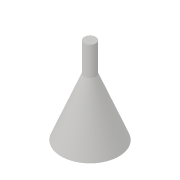
# Autodesk Inventor part: control stick
Saved by Autodesk Inventor 2018 (Build 220112000, 112)
## iProperties
Created: 2019-02-02
Part Number: control stick
Material: Generic
Document SubType Name: Modeling
Designer: ball
Density: 1 g/cm^3
Appearance: Default
Author: ball
Autodesk Inventor part; units mm, degrees
ref_plane "YZ Plane" through (0, 0, 0) normal (1, 0, 0) x (0, 1, 0)
ref_plane "XZ Plane" through (0, 0, 0) normal (0, 1, 0) x (-1, 0, 0)
ref_plane "XY Plane" through (0, 0, 0) normal (0, 0, 1) x (1, 0, 0)
sketch "Sketch1" plane through (0, 0, 0) normal (0, 0, 1) x (1, 0, 0)
  line L0 (0, 0) -> (12.7, 0)
  line L1 (0, 0) -> (0, 25.4)
  line L2 (0, 25.4) -> (2.54, 25.4)
  line L3 (2.54, 25.4) -> (12.7, 0)
  line L4 (0, 25.4) -> (2.54, 25.4)
  line L5 (2.54, 25.4) -> (2.54, 38.1)
  line L6 (2.54, 38.1) -> (0, 38.1)
  line L7 (0, 38.1) -> (0, 25.4)
  dimension "d0" = 12.7
  dimension "d1" = 25.4
  dimension "d2" = 2.54
  dimension "d3" = 12.7
  constraints: 16 end point, 3 horizontal, 2 parallel, 1 perpendicular, 1 vertical
  measures "d0" distance of L0.start L0.end
  measures "d1" distance of L0.start L1.end
  measures "d2" distance of L1.end L2.end
  measures "d3" distance of L5.end L4.end
revolve "Revolution1" add sketch "Sketch1" angle 360 about axis through (0, 0, 0) along (0, 1, 0)
body "Solid1"
